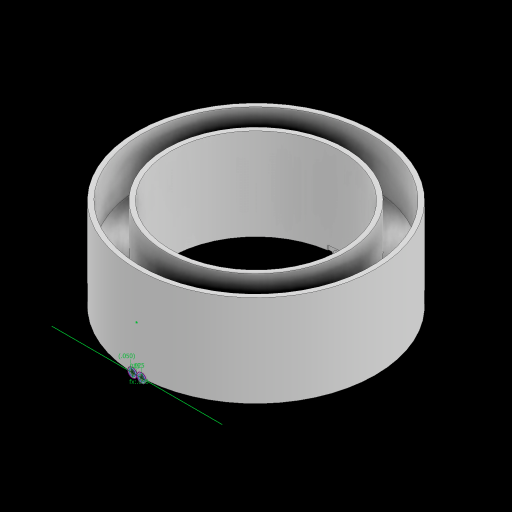
# Autodesk Inventor part: SC-1-01-Claw Attachment
Saved by Autodesk Inventor 2023 (Build 270158000, 158)
## iProperties
Created: 2023-05-15
Part Number: SC-1-01-Claw Attachment
Material: Generic
Document SubType Name: Modeling
Designer: annah
Density: 1 g/cm^3
Appearance: Default
Author: annah
Autodesk Inventor part; units mm, degrees
ref_plane "YZ Plane" through (0, 0, 0) normal (1, 0, 0) x (0, 1, 0)
ref_plane "XZ Plane" through (0, 0, 0) normal (0, 1, 0) x (-1, 0, 0)
sketch "Sketch1" plane through (0, 0, 0) normal (0, 1, 0) x (-1, 0, 0)
  circle A0 centre (0, 0) radius 12.446
  circle A1 centre (0, 0) radius 15.875
  circle A2 centre (0, 0) radius 12.7
  circle A3 centre (0, 0) radius 15.08125
  circle A4 centre (0, 0) radius 11.811
  circle A5 centre (0, 0) radius 16.51
  dimension "d2" = 24.892
  dimension "d3" = 31.75
  dimension "d6" = 25.4
  dimension "d7" = 30.1625
  dimension "d8" = 23.622
  dimension "d9" = 33.02
  constraints: 6 centre point, 5 coincident
  measures "d2" diameter of A0
  measures "d3" diameter of A1
  measures "d6" diameter of A2
  measures "d7" diameter of A3
  measures "d8" diameter of A4
  measures "d9" diameter of A5
sketch "Sketch1 outline for Extrusion2" plane through (0, 0, 0) normal (0, 1, 0) x (-1, 0, 0)
  circle A0 centre (0, 0) radius 12.446
  circle A1 centre (0, 0) radius 11.811
  circle A2 centre (0, 0) radius 16.51
  circle A3 centre (0, 0) radius 15.875
extrude "Extrusion2" add sketch "Sketch1 outline for Extrusion2" along normal blind 6.35
sketch "Sketch2" plane through (0, 0, 0) normal (0, 1, 0) x (-1, 0, 0)
  circle A0 centre (0, 0) radius 16.51
  circle A1 centre (0, 0) radius 11.811
  constraints: 2 centre point, 2 coincident
sketch "Sketch2 outline for Extrusion3" plane through (0, 0, 0) normal (0, 1, 0) x (-1, 0, 0)
  circle A0 centre (0, 0) radius 16.51
  circle A1 centre (0, 0) radius 11.811
extrude "Extrusion3" add sketch "Sketch2 outline for Extrusion3" against normal blind 6.35
ref_plane "Work Plane1" through (0, 0, 16.51) normal (0, 0, 1) x (1, 0, 0)
sketch "Sketch3" plane through (0, 0, 16.51) normal (0, 0, 1) x (1, 0, 0)
  line L0 (11.811, -6.35) -> (-11.811, -6.35)
  circle A0 centre (0.635, -6.35) radius 0.635
  circle A1 centre (-0.635, -6.35) radius 0.635
  circle A2 centre (-0.635, -6.35) radius 0.441281
  circle A3 centre (0.635, -6.35) radius 0.446106
  point P0 (0, 0)
  point P1 (0, -6.35)
  point P2 (0.188894, -6.35)
  point P3 (1.081106, -6.35)
  point P4 (-1.076281, -6.35)
  point P5 (-0.193719, -6.35)
  point P6 (0, -6.35)
  dimension "d17" = 1.27
  dimension "d14" = 0.635
  dimension "d15" = 1.27
  dimension "d16" = 0.635
  constraints: 3 centre point, 2 coincident, 2 point on line, 1 midpoint, 3 other
  measures "d14" distance of A0.centre point (0, -6.35)
  measures "d15" diameter of A0
  measures "d16" distance of point (0, -6.35) point (-0.635, -6.35)
sketch "Sketch3 outline for Extrusion4" plane through (0, 0, 16.51) normal (0, 0, 1) x (1, 0, 0)
  arc A0 (1.081106, -6.35) -> (0.188894, -6.35) centre (0.635, -6.35) ccw
  line L0 (0.188894, -6.35) -> (1.081106, -6.35)
  arc A1 (-0.193719, -6.35) -> (-1.076281, -6.35) centre (-0.635, -6.35) ccw
  line L1 (-1.076281, -6.35) -> (-0.193719, -6.35)
extrude "Extrusion4" cut sketch "Sketch3 outline for Extrusion4" against normal blind 33.02
sketch "Sketch3 outline for Extrusion5" plane through (0, 0, 16.51) normal (0, 0, 1) x (1, 0, 0)
  circle A0 centre (-0.635, -6.35) radius 0.635
  circle A1 centre (-0.635, -6.35) radius 0.441281
  circle A2 centre (0.635, -6.35) radius 0.635
  circle A3 centre (0.635, -6.35) radius 0.446106
extrude "Extrusion5" add sketch "Sketch3 outline for Extrusion5" against normal blind 33.02
sketch "Sketch4" plane through (0, 0, 0) normal (0, 1, 0) x (-1, 0, 0)
  circle A0 centre (0, 0) radius 11.811
  line L0 (0, -11.811) -> (-1.75015, -11.811)
  line L1 (-1.75015, -11.811) -> (-1.75015, 11.811)
  line L2 (-1.75015, 11.811) -> (0, 11.811)
  line L3 (0, 11.811) -> (0, -11.811)
  line L4 (0, 11.811) -> (1.734243, 11.811)
  line L5 (1.734243, 11.811) -> (1.734243, -11.811)
  line L6 (1.734243, -11.811) -> (0, -11.811)
  line L7 (0, -11.811) -> (0, 11.811)
  line L8 (1.759637, -13.430634) -> (-1.759637, -13.430634)
  line L9 (-1.759637, -13.430634) -> (-1.759637, -14.890366)
  line L10 (-1.759637, -14.890366) -> (1.759637, -14.890366)
  line L11 (1.759637, -14.890366) -> (1.759637, -13.430634)
  line L12 (0, -11.811) -> (0, -16.51)
  line L13 (1.759637, -13.430634) -> (-1.759637, -14.890366) construction
  line L14 (-1.759637, -13.430634) -> (1.759637, -14.890366) construction
  circle A1 centre (0, 0) radius 16.51
  line L15 (1.762099, 14.8844) -> (-1.762099, 14.8844)
  line L16 (-1.762099, 14.8844) -> (-1.762099, 13.4366)
  line L17 (-1.762099, 13.4366) -> (1.762099, 13.4366)
  line L18 (1.762099, 13.4366) -> (1.762099, 14.8844)
  line L19 (1.762099, 14.8844) -> (-1.762099, 13.4366) construction
  line L20 (-1.762099, 14.8844) -> (1.762099, 13.4366) construction
  line L21 (0, 16.51) -> (0, 11.811)
  point P0 (0, -14.1605)
  point P1 (0, 14.1605)
  point P2 (0, 14.1605)
  dimension "d22" = 1.61963
  dimension "d23" = 1.61963
  dimension "d24" = 0
  dimension "d25" = 3.81
  dimension "d26" = 3.81
  dimension "d27" = 3.81
  dimension "d28" = 3.81
  dimension "d29" = 1.6256
  dimension "d30" = 1.6256
  constraints: 40 end point, 8 parallel, 6 midpoint, 4 horizontal, 4 perpendicular, 1 point on line, 1 vertical alignment, 1 other
  measures "d23" distance edge to line of A1 L10
  measures "d24" distance of point (0, 14.161) point (0, 14.161)
  measures "d25" distance of L8.end L10.end
  measures "d26" distance of L8.start L9.end
  measures "d27" distance of L15.end L17.end
  measures "d28" distance of L15.start L16.end
  measures "d29" distance from line of L2.end L17
  measures "d30" distance from line of L21.start L15
sketch "Sketch5" plane through (0, -6.35, 0) normal (0, -1, 0) x (1, 0, 0)
  line L0 (0, -11.811) -> (-1.75015, -11.811)
  line L1 (-1.75015, -11.811) -> (-1.75015, 11.811)
  line L2 (-1.75015, 11.811) -> (0, 11.811)
  line L3 (0, 11.811) -> (0, -11.811)
  line L4 (0, 11.811) -> (1.734243, 11.811)
  line L5 (1.734243, 11.811) -> (1.734243, -11.811)
  line L6 (1.734243, -11.811) -> (0, -11.811)
  line L7 (0, -11.811) -> (0, 11.811)
  line L8 (1.759637, -13.430634) -> (-1.759637, -13.430634)
  line L9 (-1.759637, -13.430634) -> (-1.759637, -14.890366)
  line L10 (-1.759637, -14.890366) -> (1.759637, -14.890366)
  line L11 (1.759637, -14.890366) -> (1.759637, -13.430634)
  line L12 (0, -11.811) -> (0, -16.51)
  line L13 (1.759637, -13.430634) -> (-1.759637, -14.890366) construction
  line L14 (-1.759637, -13.430634) -> (1.759637, -14.890366) construction
  line L15 (1.762099, 14.8844) -> (-1.762099, 14.8844)
  line L16 (-1.762099, 14.8844) -> (-1.762099, 13.4366)
  line L17 (-1.762099, 13.4366) -> (1.762099, 13.4366)
  line L18 (1.762099, 13.4366) -> (1.762099, 14.8844)
  line L19 (1.762099, 14.8844) -> (-1.762099, 13.4366) construction
  line L20 (-1.762099, 14.8844) -> (1.762099, 13.4366) construction
  line L21 (0, 16.51) -> (0, 11.811)
  point P0 (0, 0)
  point P1 (0, 0)
  point P2 (0, 0)
  point P3 (0, -14.1605)
  point P4 (0, 0)
  point P5 (0, 14.1605)
  point P6 (0, 14.1605)
  dimension "d33" = 0
  dimension "d34" = 3.81
  dimension "d35" = 3.81
  dimension "d36" = 3.81
  dimension "d37" = 3.81
  dimension "d38" = 1.6256
  dimension "d39" = 1.6256
  constraints: 44 end point, 8 parallel, 6 midpoint, 4 horizontal, 4 perpendicular, 1 point on line
  measures "d33" distance of point (0, 14.161) point (0, 14.161)
  measures "d34" distance of L8.end L11.start
  measures "d35" distance of L8.start L10.start
  measures "d36" distance of L15.end L17.end
  measures "d37" distance of L18.end L17.start
  measures "d38" distance from line of L2.end L17
  measures "d39" distance from line of L21.start L15
sketch "Sketch5 outline for Extrusion7" plane through (0, -6.35, 0) normal (0, -1, 0) x (1, 0, 0)
  line L0 (-1.759637, -13.430634) -> (-1.759637, -14.890366)
  line L1 (1.759637, -13.430634) -> (-1.759637, -13.430634)
  line L2 (1.759637, -14.890366) -> (1.759637, -13.430634)
  line L3 (-1.759637, -14.890366) -> (1.759637, -14.890366)
  line L4 (-1.762099, 14.8844) -> (-1.762099, 13.4366)
  line L5 (1.762099, 14.8844) -> (-1.762099, 14.8844)
  line L6 (1.762099, 13.4366) -> (1.762099, 14.8844)
  line L7 (-1.762099, 13.4366) -> (1.762099, 13.4366)
  line L8 (-1.75015, -11.811) -> (1.734243, -11.811)
  line L9 (1.734243, -11.811) -> (1.734243, 11.811)
  line L10 (1.734243, 11.811) -> (-1.75015, 11.811)
  line L11 (-1.75015, 11.811) -> (-1.75015, -11.811)
extrude "Extrusion7" cut sketch "Sketch5 outline for Extrusion7" along normal mid plane 1.27
equation "\"d15\" = 2 * d14"
body "Solid2"
